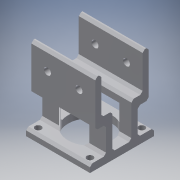
# Autodesk Inventor part: MSUP
Saved by Autodesk Inventor 2016 (Build 200138000, 138)
## iProperties
Created: 2017-07-13
Part Number: MSUP
Material: PC/ABS Plastic
Document SubType Name: Modeling
Designer: ludwi
Density: 0.357273 g/cm^3
Appearance: Smooth - White
Author: ludwi
Autodesk Inventor part; units mm, degrees
ref_plane "YZ Plane" through (0, 0, 0) normal (1, 0, 0) x (0, 1, 0)
ref_plane "XZ Plane" through (0, 0, 0) normal (0, 1, 0) x (-1, 0, 0)
ref_plane "XY Plane" through (0, 0, 0) normal (0, 0, 1) x (1, 0, 0)
sketch "Sketch8" plane through (0, 0, 0) normal (1, 0, 0) x (0, 1, 0)
  line L0 (4.5, 60.5) -> (11.541, 60.5) construction
  line L1 (11.541, 60.5) -> (11.541, 69.5) construction
  line L2 (11.541, 69.5) -> (16, 69.5) construction
  line L3 (16, 69.5) -> (18, 67.5) construction
  line L4 (18, 67.5) -> (18, 39.5) construction
  line L5 (18, 39.5) -> (16, 37.5) construction
  line L6 (16, 37.5) -> (12, 37.5) construction
  line L7 (12, 37.5) -> (12, 46.5) construction
  line L8 (12, 46.5) -> (4.5, 46.5) construction
  line L9 (4.5, 46.5) -> (4.5, 60.5) construction
  line L10 (-11.541, 60.5) -> (-4.5, 60.5) construction
  line L11 (-4.5, 60.5) -> (-4.5, 46.5) construction
  line L12 (-4.5, 46.5) -> (-12, 46.5) construction
  line L13 (-12, 46.5) -> (-12, 37.5) construction
  line L14 (-12, 37.5) -> (-16, 37.5) construction
  line L15 (-16, 37.5) -> (-18, 39.5) construction
  line L16 (-18, 39.5) -> (-18, 67.5) construction
  line L17 (-18, 67.5) -> (-16, 69.5) construction
  line L18 (-16, 69.5) -> (-11.541, 69.5) construction
  line L19 (-11.541, 69.5) -> (-11.541, 60.5) construction
  line L20 (-3.125, -5) -> (3.125, -5) construction
  line L21 (3.125, -5) -> (3.125, 0) construction
  line L22 (3.125, 0) -> (-3.125, 0) construction
  line L23 (-3.125, 0) -> (-3.125, -5) construction
  line L24 (19, 2) -> (19, 0) construction
  line L25 (19, 0) -> (27.75, 0) construction
  line L26 (27.75, 0) -> (27.75, -80) construction
  line L27 (27.75, -80) -> (-27.75, -80) construction
  line L28 (-27.75, -80) -> (-27.75, 0) construction
  line L29 (-27.75, 0) -> (-19, 0) construction
  line L30 (-19, 0) -> (-19, 2) construction
  line L31 (-19, 2) -> (-3.125, 2) construction
  line L32 (-3.125, 2) -> (-3.125, 22) construction
  line L33 (-3.125, 22) -> (3.125, 22) construction
  line L34 (3.125, 22) -> (3.125, 2) construction
  line L35 (3.125, 2) -> (19, 2) construction
  line L36 (27.75, 0) -> (-27.75, 0) construction
  line L37 (-27.75, 0) -> (-27.75, 6.5)
  line L38 (-27.75, 6.5) -> (27.75, 6.5) construction
  line L39 (27.75, 0) -> (27.75, 6.5) construction
  line L40 (27.75, 6.5) -> (19, 6.5) construction
  line L41 (27.75, 6.5) -> (18, 6.5) construction
  line L42 (18, 6.5) -> (18, 69.5) construction
  line L43 (18, 69.5) -> (27.75, 69.5) construction
  line L44 (27.75, 69.5) -> (27.75, 6.5) construction
  line L45 (-27.75, 6.5) -> (-18, 6.5) construction
  line L46 (-18, 6.5) -> (-18, 69.5) construction
  line L47 (-18, 69.5) -> (-27.75, 69.5) construction
  line L48 (-27.75, 69.5) -> (-27.75, 6.5) construction
  line L49 (7.7602, 6.5) -> (14.2602, 6.5) construction
  line L50 (14.2602, 6.5) -> (14.2602, 36) construction
  line L51 (14.2602, 36) -> (7.7602, 36) construction
  line L52 (7.7602, 36) -> (7.7602, 6.5) construction
  line L53 (-15.5, 6.5) -> (-9, 6.5)
  line L54 (-9, 6.5) -> (-9, 36)
  line L55 (-9, 36) -> (-15.5, 36)
  line L56 (-15.5, 36) -> (-15.5, 6.5)
  line L57 (-18, 69.5) -> (-24.5, 69.5)
  line L58 (-24.5, 69.5) -> (-24.5, 29.5)
  line L59 (-24.5, 29.5) -> (-18, 29.5)
  line L60 (-18, 29.5) -> (-18, 69.5)
  line L61 (18, 69.5) -> (24.5, 69.5) construction
  line L62 (24.5, 69.5) -> (24.5, 29.5) construction
  line L63 (24.5, 29.5) -> (18, 29.5) construction
  line L64 (18, 29.5) -> (18, 69.5) construction
  line L65 (14.2602, 36) -> (18, 36) construction
  line L66 (18, 36) -> (18, 29.5) construction
  line L67 (18, 29.5) -> (14.2602, 29.5) construction
  line L68 (14.2602, 29.5) -> (14.2602, 36) construction
  line L69 (-15.5, 36) -> (-18, 36)
  line L70 (-18, 36) -> (-18, 29.5)
  line L71 (-18, 29.5) -> (-15.5, 29.5)
  line L72 (-15.5, 29.5) -> (-15.5, 36)
  line L73 (0, 6.5) -> (0, 0)
  line L74 (-27.75, 6.5) -> (-9, 6.5)
  line L75 (-9, 6.5) -> (-9, 0)
  line L76 (-9, 0) -> (-27.75, 0)
  line L77 (-27.75, 0) -> (-27.75, 6.5)
  point P0 (18, 38)
  point P1 (-9, 3.25)
  point P2 (-9, 21.25)
  dimension "d46" = 40
  dimension "d47" = 6.5
  dimension "d48" = 6.5
  dimension "d49" = 6.5
  dimension "d50" = 2.5
  dimension "d51" = 6.5
  constraints: 156 end point, 26 horizontal, 19 parallel, 17 vertical, 11 perpendicular, 5 equal length, 5 midpoint, 4 point on line, 2 vertical alignment, 1 horizontal alignment, 40 other
  measures "d46" distance of L57.end L58.end
  measures "d47" distance of L58.end L59.end
  measures "d48" distance of L28.end L37.end
  measures "d49" distance of L54.end L55.end
  measures "d50" distance of L55.end L69.end
  measures "d51" distance of L69.end L59.end
ref_plane "Work Plane5" through (27.75, -25.25, -80) normal (1, 0, 0) x (0, 1, 0)
ref_plane "Work Plane6" through (-27.75, -25.25, -80) normal (-1, 0, 0) x (0, 0, 1)
extrude "Extrusion7" add sketch "Sketch8" against normal up to surface (55.5 mm away) from surface at 27.75
sketch "Sketch14" plane through (-27.75, -27.75, 6.5) normal (0, 0, 1) x (1, 0, 0)
  circle A0 centre (5.25, 5.25) radius 2.75 projected
  circle A1 centre (50.25, 5.25) radius 2.75 projected
  point P0 (27.75, 27.75)
extrude "Extrusion12" cut sketch "Sketch14" against normal through all
sketch "Sketch15" plane through (27.75, -9, 0) normal (0, 0, -1) x (-1, 0, 0)
  circle A0 centre (27.75, 9) radius 19 projected
extrude "Extrusion13" cut sketch "Sketch15" against normal up to surface (29.5 mm away)
sketch "Sketch16" plane through (-27.75, -24.5, 29.5) normal (0, -1, 0) x (1, 0, 0)
  circle A0 centre (41.45, 24) radius 3 projected
  circle A1 centre (14.05, 24) radius 3 projected
  point P0 (27.75, -29.5)
extrude "Extrusion14" cut sketch "Sketch16" against normal through all
chamfer "Chamfer6" distance 2 angle 45 12 edges at (0, -24.5, 69.5) (0, -18, 69.5) (0, -24.5, 29.5) (0, -27.75, 6.5) (-22.2416, -9, 0) (22.2416, -9, 0) (0, -9, 36) (0, -9, 29.5) (-19.3693, -15.5, 6.5) (19.3693, -15.5, 6.5) (-19.3693, -15.5, 29.5) (19.3693, -15.5, 29.5)
body "Solid3"
